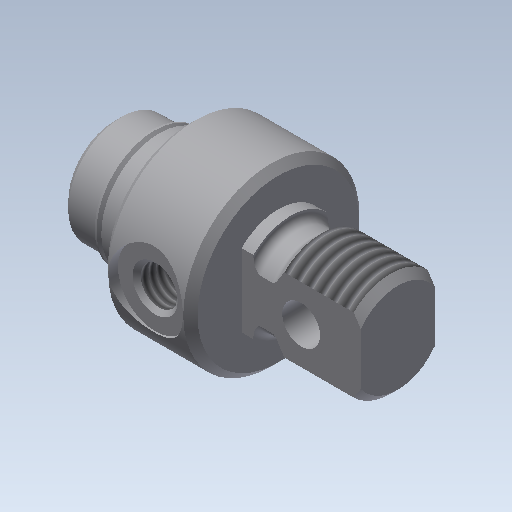
# Autodesk Inventor part: 01P0000_rear_head
Saved by Autodesk Inventor 2020 (Build 240168000, 168)
## iProperties
Created: 2020-01-07
Part Number: 01P0000_rear_head
Material: Generic
Catalog Web Link: www.cadenas.de
Description: Rear Head-Original Line - Standard Air Cylinders
Vendor: BIMBA
Document SubType Name: Modeling
Designer: psadmin
Manufacturer: BIMBA
Mass: 3.86005 g
Surface Area: 22.3376 cm^2
Volume: 3.86005 cm^3
Density: 1 g/cm^3
Appearance: PSOLRGB-211-211-211
Category: PARTsolutions
Company: BIMBA
PSOL_IDENT_0: {$CADENAS_DATA\23d-libs\bimba\bimba_brand\bimba_imperial\bimba_full_line\original_line_cylinders\sta
PSOL_IDENT_1: ndard_air_cylinders\rear_head.prj},239 {VTYP=3D},{NB=01P0000_rear_head},{LINA=01P0000_rear_head},{NN=
PSOL_IDENT_2: Rear Head},{DATE=23.12.2019 10:40:48},{GEOMDATE=15.10.2019 12:00:43},{VERSION=},{LINEID=20},{WBVAR=M
PSOL_IDENT_3: NT,ACTING,DER,Q,T1,T2,T3,T4,TRIM,Y,K,MB,CUSH,FBON},{WBNUMERIC=TRIM,MB,CUSH}  {NB=01P0000_rear_head},
PSOL_IDENT_4: {LINA=01P0000_rear_head},{KT=DUMMY},{PN=01P0000},{BORE=0.43750},{BOREPN=01},{MNT=P},{MNTALG='' , 'Fr
PSOL_IDENT_5: ont Nose' , 'P' , 'Rear Pivot' , 'DX' , 'Double End' , 'BR' , 'Rear Block' , 'BRT' , 'Rear Trunnion'
PSOL_IDENT_6: },{ACTING=},{ACTINGALG= '' , 'Single Acting' },{DER=},{DERALG= '' , 'Standard' },{Q=},{T1=},{T2=},{T
PSOL_IDENT_7: 3=},{T4=},{TRIM=0},{Y=},{K=},{KALG= '', 'without K', 'K', 'with K' },{MB=0},{A1=1.1880},{A1N=0.5000}
PSOL_IDENT_8: ,{A1P=1.1880},{A1B=0.8120},{A1S=0.0000},{A2=0.188},{A2N=0.1880},{A3=0.0200},{D1=0.7380},{D1N=0.4855}
PSOL_IDENT_9: ,{D1P=0.7380},{D1B=0.4855},{D2=0.4465},{C1=0.0300},{C2=0.0300},{NDM=0.1900},{TAB=UNF},{NDMDP=0.2000}
PSOL_IDENT_10: ,{D3=0.1600},{A4=0.1880},{A5=0.3700},{D4=0.0000},{A6=0.0000},{A7=0.5000},{A8=0.1250},{D5=0.4855},{D6=
PSOL_IDENT_11: 0.1875},{A9=0.6250},{NDM2=0.4375},{TAB2=UNF},{C11=0.0300},{C22=0.0000},{C33=0.0300},{C44=0.0300},{A1
PSOL_IDENT_12: 0=0.3095},{A11=0.0000},{NDM3=0.1900},{NDM3N=0.1900},{NDM3B=0.1900},{TAB3=UNF},{TAB3N=UNF},{TAB3B=UNF
PSOL_IDENT_13: },{A12=0.5},{A12N=0.5000},{A12B=0.4680},{A13=0.9380},{D7=0.1590},{D8=0.4350},{A14=0.0500},{A15=0.077
PSOL_IDENT_14: 5},{D9=0.3600},{R1=0.0315},{X1=0.0000},{X2=0.0000},{CX=0.0000},{CC=0.0000},{CON=1},{S1=0.7500},{DB=0
PSOL_IDENT_15: .1562},{X1B=0.2500},{X2B=0.0620},{A8B=0.1250},{A9B=0.5620},{MODEL=1},{NDM4=0.1640},{TAB4=UNC},{NDM4D
PSOL_IDENT_16: P=0.2500},{BC=0.7500},{B1=0.5620},{B2=0.2500},{B3=0.3740},{ON=0},{ON2=1},{G1=0.0000},{G2=0.0000},{G3=
PSOL_IDENT_17: 0.0000},{G4=0.0000},{GD=0.0000},{G5=0.0000},{G6=0.0000},{RON=0},{H1=0.0000},{H2=0.0000},{H3=0.0000},
PSOL_IDENT_18: {H4=0.0000},{H5=0.0000},{H6=0.0000},{F=0.0000},{PNUT=0.7380},{CUSH=0},{CC11=0.000},{CC111=0.0000},{C
PSOL_IDENT_19: C22=0.0000},{CC33=0.0000},{CC44=0.0000},{CC55=0.0000},{CD1=0.0000},{CD2=0.0000},{CD3=0.0000},{CNDM3=
PSOL_IDENT_20: 0.0000},{CTAB3=0.0000},{OLEN=0.9380},{OD=0.2185},{STDIS=0.0000},{STDIS1=0.0000},{BUSHCON=D-8597},{BU
PSOL_IDENT_21: SHL=0.3120},{FBON=0},{LCD=0.0000}
NN: Rear Head
NT: Original Line - Standard Air Cylinders
NB: 01P0000_rear_head
NBSYN: $PN._rear_head
LINA: 01P0000_rear_head
PN: 01P0000
BORE: 0.4375
BOREPN: 01
MNT: Rear Pivot
MNTALG: '' , 'Front Nose' , 'P' , 'Rear Pivot' , 'DX' , 'Double End' , 'BR' , 'Rear Block' , 'BRT' , 'Rear Trunnion'
ACTING: Single Acting
DER: Standard
Q: Without Side Ported Rear Head
T1: without T1
T2: without T2
T3: without T3
T4: without T4
TRIM: 0
Y: without Pivot Bushing
K: without K
MB: 0
A1N: 0.5
A1P: 1.188
A1B: 0.812
A1S: 0
A2N: 0.188
A3: 0.02
D1N: 0.4855
D1P: 0.738
D1B: 0.4855
D2: 0.4465
C1: 0.03
C2: 0.03
TAB: UNF
NDMDP: 0.2
D3: 0.16
A4: 0.188
A5: 0.37
D4: 0
A6: 0
A7: 0.5
A8: 0.125
D5: 0.4855
D6: 0.1875
A9: 0.625
NDM2: 0.4375
TAB2: UNF
C11: 0.03
C22: 0
C33: 0.03
C44: 0.03
A10: 0.3095
A11: 0
NDM3N: 0.19
NDM3B: 0.19
TAB3N: UNF
TAB3B: UNF
A12N: 0.5
A12B: 0.468
A13: 0.938
D7: 0.159
D8: 0.435
A14: 0.05
A15: 0.0775
D9: 0.36
R1: 0.0315
X1: 0
X2: 0
CX: 0
CC: 0
S1: 0.75
DB: 0.1562
X1B: 0.25
X2B: 0.062
A8B: 0.125
A9B: 0.562
NDM4: 0.164
TAB4: UNC
NDM4DP: 0.25
BC: 0.75
B1: 0.562
B2: 0.25
B3: 0.374
G1: 0
G2: 0
G3: 0
G4: 0
GD: 0
G5: 0
G6: 0
H2: 0
H3: 0
F: 0
CUSH: 0
CC111: 0
CC22: 0
CC33: 0
CC44: 0
CC55: 0
CD1: 0
CD2: 0
CD3: 0
CNDM3: 0
CTAB3: 0.0000
OD: 0.2185
STDIS1: 0
BUSHCON: D-8597
BUSHL: 0.312
FBON: 0
LCD: 0
SUPPLIER: BIMBA
ARTICLENO: 01P0000_rear_head
BOMINFO: 01P0000_rear_head
CREATOR: CADENAS GmbH
Title: 01P0000_rear_head
Author: Cadenas PARTsolutions
Comments: Original Line - Standard Air Cylinders
Autodesk Inventor part; units mm, degrees
ref_plane "YZ Plane" through (0, 0, 0) normal (1, 0, 0) x (0, 1, 0)
ref_plane "XZ Plane" through (0, 0, 0) normal (0, 1, 0) x (-1, 0, 0)
ref_plane "XY Plane" through (0, 0, 0) normal (0, 0, 1) x (1, 0, 0)
sketch "Sketch_8" plane through (0, 0, 0) normal (0, 0, 1) x (1, 0, 0)
  line L0 (17.4752, 0) -> (0, 0)
  line L1 (0, 0) -> (0, 4.9085)
  line L2 (0, 4.9085) -> (0.762, 5.6706)
  line L3 (0.762, 5.6706) -> (3.7592, 5.6706)
  line L4 (3.7592, 5.6706) -> (4.2672, 5.1626)
  line L5 (4.2672, 5.1626) -> (4.7752, 5.1626)
  line L6 (4.7752, 5.1626) -> (4.7752, 6.1659)
  line L7 (4.7752, 6.1659) -> (7.9502, 6.1659)
  line L8 (7.9502, 6.1659) -> (7.9502, 8.6106)
  line L9 (7.9502, 8.6106) -> (8.7122, 9.3726)
  line L10 (8.7122, 9.3726) -> (16.7132, 9.3726)
  line L11 (16.7132, 9.3726) -> (17.4752, 8.6106)
  line L12 (17.4752, 8.6106) -> (17.4752, 0)
  line L13 (17.4752, 0) -> (0, 0)
  constraints: 28 end point
revolve "Revolution1" add sketch "Sketch_8" angle 360 about axis through (17.4752, 0, 0) along (1, 0, 0)
sketch "Sketch_15" plane through (0, 0, 0) normal (0, 0, 1) x (1, 0, 0)
  line L0 (30.1752, 0) -> (17.4752, 0)
  line L1 (17.4752, 0) -> (17.4752, 5.5245)
  line L2 (17.4752, 5.5245) -> (18.7452, 5.5245)
  line L3 (18.7452, 5.5245) -> (18.7452, 5.3721)
  arc A0 (18.7452, 5.3721) -> (19.5453, 4.572) centre (19.5453, 5.3721) ccw
  line L4 (19.5453, 4.572) -> (20.7137, 4.572)
  arc A1 (20.7137, 4.572) -> (21.2166, 4.7498) centre (20.7137, 5.3721) ccw
  line L5 (21.2166, 4.7498) -> (21.2795, 4.8006)
  line L6 (21.2795, 4.8006) -> (22.0351, 5.5563)
  line L7 (22.0351, 5.5563) -> (29.4196, 5.5563)
  line L8 (29.4196, 5.5563) -> (30.1752, 4.8006)
  line L9 (30.1752, 4.8006) -> (30.1752, 0)
  line L10 (30.1752, 0) -> (17.4752, 0)
  constraints: 22 end point, 4 point on circle, 2 centre point
revolve "Revolution2" add sketch "Sketch_15" angle 360 about axis through (30.1752, 0, 0) along (1, 0, 0)
thread "Thread1" size "7/16-20 UNF" class "2A" standard "ANSI Unified Screw Threads" full length
sketch "Sketch_9" plane through (30.1752, 0, 0) normal (1, 0, 0) x (0, 0, -1)
  line L0 (-18.7452, -37.4904) -> (18.7452, -37.4904)
  line L1 (18.7452, -37.4904) -> (18.7452, 37.4904)
  line L2 (18.7452, 37.4904) -> (-18.7452, 37.4904)
  line L3 (-18.7452, 37.4904) -> (-18.7452, -37.4904)
  line L4 (-3.9306, -18.7452) -> (3.9306, -18.7452)
  line L5 (3.9306, -18.7452) -> (3.9306, 18.7452)
  line L6 (3.9306, 18.7452) -> (-3.9306, 18.7452)
  line L7 (-3.9306, 18.7452) -> (-3.9306, -18.7452)
  constraints: 16 end point
extrude "Extrusion1" cut sketch "Sketch_9" against normal blind 12.7
sketch "Sketch4" plane through (0, 0, 0) normal (-1, 0, 0) x (0, 0, 1)
  point P0 (0, 0)
hole "Hole1" at (0, 0, 0) direction (1, 0, 0) diameter 4.7625 depth 17.4625 tip angle 120
sketch "Sketch_16" plane through (0, 0, 0) normal (0, 1, 0) x (-1, 0, 0)
  line L0 (-12.7, 9.3726) -> (-12.7, 0)
  line L1 (-12.7, 0) -> (-14.6837, 0)
  line L2 (-14.6837, 0) -> (-14.6837, 7.9273)
  line L3 (-14.6837, 7.9273) -> (-15.113, 8.3566)
  line L4 (-15.113, 8.3566) -> (-16.6624, 8.3566)
  line L5 (-16.6624, 8.3566) -> (-16.6624, 9.3726)
  line L6 (-16.6624, 9.3726) -> (-12.7, 9.3726)
  line L7 (-12.7, 9.3726) -> (-12.7, 0)
  constraints: 16 end point
revolve "Revolution3" cut sketch "Sketch_16" angle 360 about axis through (12.7, 0, 9.3726) along (0, 0, 1)
thread "Thread2" size "10-32 UNF" class "2B" standard "ANSI Unified Screw Threads" length 5.5461
sketch "Sketch_24" plane through (0, 0, 0) normal (0, 0, 1) x (1, 0, 0)
  line L0 (4.7752, 0) -> (4.2672, 0)
  line L1 (4.0665, 6.1659) -> (4.0665, 6.0817)
  line L2 (4.0665, 6.0817) -> (4.6636, 5.4846)
  arc A0 (4.6636, 5.305) -> (4.6636, 5.4846) centre (4.5738, 5.3948) ccw
  line L3 (4.6636, 5.305) -> (4.5212, 5.1626)
  line L4 (4.5212, 5.1626) -> (4.2672, 5.1626)
  line L5 (4.2672, 5.1626) -> (4.2672, 4.9085)
  line L6 (4.2672, 4.9085) -> (4.7752, 4.9085)
  line L7 (4.7752, 4.9085) -> (4.7752, 5.6603)
  line L8 (4.7752, 5.6603) -> (4.2697, 6.1659)
  line L9 (4.2697, 6.1659) -> (4.0665, 6.1659)
  constraints: 20 end point, 2 point on circle, 1 centre point
revolve "Revolution4" add sketch "Sketch_24" angle 360 about axis through (4.7752, 0, 0) along (1, 0, 0)
sketch "Sketch_43" plane through (0, 0, 0) normal (0, 0, 1) x (1, 0, 0)
  circle A0 centre (23.8252, 0) radius 2.0193
  constraints: 1 centre point
extrude "Extrusion2" cut sketch "Sketch_43" along normal mid plane 11.7919
ref_plane "1_XY" through (18.7452, 0, 0) normal (1, 0, 0) x (0, 0, -1)
ref_plane "1_YZ" through (18.7452, 0, 0) normal (0, 0, -1) x (0, 1, 0)
ref_plane "1_ZX" through (18.7452, 0, 0) normal (0, 1, 0) x (1, 0, 0)
ref_plane "c1_XY" through (17.4752, 5.5245, 0) normal (0, 0, 1) x (1, 0, 0)
ref_plane "c1_YZ" through (17.4752, 5.5245, 0) normal (1, 0, 0) x (0, 1, 0)
ref_plane "c1_ZX" through (17.4752, 5.5245, 0) normal (0, 1, 0) x (0, 0, 1)
ref_plane "c2_XY" through (17.4752, -5.5245, 0) normal (0, 0, 1) x (1, 0, 0)
ref_plane "c2_YZ" through (17.4752, -5.5245, 0) normal (1, 0, 0) x (0, 1, 0)
ref_plane "c2_ZX" through (17.4752, -5.5245, 0) normal (0, 1, 0) x (0, 0, 1)
ref_plane "cc1_XY" through (17.4752, 0, 0) normal (0, 0, 1) x (1, 0, 0)
ref_plane "cc1_YZ" through (17.4752, 0, 0) normal (1, 0, 0) x (0, 1, 0)
ref_plane "cc1_ZX" through (17.4752, 0, 0) normal (0, 1, 0) x (0, 0, 1)
ref_plane "cc2_XY" through (18.7452, 0, 0) normal (0, 0, 1) x (1, 0, 0)
ref_plane "cc2_YZ" through (18.7452, 0, 0) normal (1, 0, 0) x (0, 1, 0)
ref_plane "cc2_ZX" through (18.7452, 0, 0) normal (0, 1, 0) x (0, 0, 1)
ref_plane "lovra1_XY" through (25.4, 0, 0) normal (1, 0, 0) x (0, 0, -1)
ref_plane "lovra1_YZ" through (25.4, 0, 0) normal (0, 0, -1) x (0, 1, 0)
ref_plane "lovra1_ZX" through (25.4, 0, 0) normal (0, 1, 0) x (1, 0, 0)
ref_plane "lovra2_XY" through (25.4, 4.699, 0) normal (1, 0, 0) x (0, 0, -1)
ref_plane "lovra2_YZ" through (25.4, 4.699, 0) normal (0, 0, -1) x (0, 1, 0)
ref_plane "lovra2_ZX" through (25.4, 4.699, 0) normal (0, 1, 0) x (1, 0, 0)
ref_plane "lovra21_XY" through (0, 0, 5.2705) normal (1, 0, 0) x (0, 0, -1)
ref_plane "lovra21_YZ" through (0, 0, 5.2705) normal (0, 0, -1) x (0, 1, 0)
ref_plane "lovra21_ZX" through (0, 0, 5.2705) normal (0, 1, 0) x (1, 0, 0)
ref_plane "lovra22_XY" through (0, 0, -5.2705) normal (1, 0, 0) x (0, 0, -1)
ref_plane "lovra22_YZ" through (0, 0, -5.2705) normal (0, 0, -1) x (0, 1, 0)
ref_plane "lovra22_ZX" through (0, 0, -5.2705) normal (0, 1, 0) x (1, 0, 0)
ref_plane "lovra3_XY" through (25.4, -4.699, 0) normal (1, 0, 0) x (0, 0, -1)
ref_plane "lovra3_YZ" through (25.4, -4.699, 0) normal (0, 0, -1) x (0, 1, 0)
ref_plane "lovra3_ZX" through (25.4, -4.699, 0) normal (0, 1, 0) x (1, 0, 0)
ref_plane "olen_XY" through (23.8252, 0, 0) normal (1, 0, 0) x (0, 0, -1)
ref_plane "olen_YZ" through (23.8252, 0, 0) normal (0, 0, -1) x (0, 1, 0)
ref_plane "olen_ZX" through (23.8252, 0, 0) normal (0, 1, 0) x (1, 0, 0)
ref_plane "p1_XY" through (30.1752, 0, 3.9306) normal (1, 0, 0) x (0, 0, -1)
ref_plane "p1_YZ" through (30.1752, 0, 3.9306) normal (0, 0, -1) x (0, 1, 0)
ref_plane "p1_ZX" through (30.1752, 0, 3.9306) normal (0, 1, 0) x (1, 0, 0)
ref_plane "p2_XY" through (30.1752, 0, -3.9306) normal (1, 0, 0) x (0, 0, -1)
ref_plane "p2_YZ" through (30.1752, 0, -3.9306) normal (0, 0, -1) x (0, 1, 0)
ref_plane "p2_ZX" through (30.1752, 0, -3.9306) normal (0, 1, 0) x (1, 0, 0)
ref_plane "port_XY" through (12.7, 0, 0) normal (0, 0, 1) x (1, 0, 0)
ref_plane "port_YZ" through (12.7, 0, 0) normal (1, 0, 0) x (0, 1, 0)
ref_plane "port_ZX" through (12.7, 0, 0) normal (0, 1, 0) x (0, 0, 1)
ref_plane "port2_XY" through (30.1752, 0, 0) normal (1, 0, 0) x (0, 0, -1)
ref_plane "port2_YZ" through (30.1752, 0, 0) normal (0, 0, -1) x (0, 1, 0)
ref_plane "port2_ZX" through (30.1752, 0, 0) normal (0, 1, 0) x (1, 0, 0)
ref_plane "thd1_XY" through (30.1752, 0, 5.5563) normal (1, 0, 0) x (0, 0, -1)
ref_plane "thd1_YZ" through (30.1752, 0, 5.5563) normal (0, 0, -1) x (0, 1, 0)
ref_plane "thd1_ZX" through (30.1752, 0, 5.5563) normal (0, 1, 0) x (1, 0, 0)
ref_plane "thd2_XY" through (30.1752, 0, -5.5563) normal (1, 0, 0) x (0, 0, -1)
ref_plane "thd2_YZ" through (30.1752, 0, -5.5563) normal (0, 0, -1) x (0, 1, 0)
ref_plane "thd2_ZX" through (30.1752, 0, -5.5563) normal (0, 1, 0) x (1, 0, 0)
ref_plane "to_mounting_bracket_XY" through (17.4752, 0, 0) normal (1, 0, 0) x (0, 0, -1)
ref_plane "to_mounting_bracket_YZ" through (17.4752, 0, 0) normal (0, 0, -1) x (0, 1, 0)
ref_plane "to_mounting_bracket_ZX" through (17.4752, 0, 0) normal (0, 1, 0) x (1, 0, 0)
ref_plane "to_nut_XY" through (18.7452, 0, 0) normal (1, 0, 0) x (0, 0, -1)
ref_plane "to_nut_YZ" through (18.7452, 0, 0) normal (0, 0, -1) x (0, 1, 0)
ref_plane "to_nut_ZX" through (18.7452, 0, 0) normal (0, 1, 0) x (1, 0, 0)
ref_plane "to_pin_XY" through (23.8252, 0, 0) normal (0, 0, 1) x (1, 0, 0)
ref_plane "to_pin_YZ" through (23.8252, 0, 0) normal (1, 0, 0) x (0, 1, 0)
ref_plane "to_pin_ZX" through (23.8252, 0, 0) normal (0, 1, 0) x (0, 0, 1)
ref_plane "to_screw_XY" through (12.7, 0, 0) normal (0, 1, 0) x (1, 0, 0)
ref_plane "to_screw_YZ" through (12.7, 0, 0) normal (1, 0, 0) x (0, 0, -1)
ref_plane "to_screw_ZX" through (12.7, 0, 0) normal (0, 0, -1) x (0, 1, 0)
ref_plane "to_tube_XY" through (4.2672, 0, 0) normal (1, 0, 0) x (0, 0, -1)
ref_plane "to_tube_YZ" through (4.2672, 0, 0) normal (0, 0, -1) x (0, 1, 0)
ref_plane "to_tube_ZX" through (4.2672, 0, 0) normal (0, 1, 0) x (1, 0, 0)
body "Solid1"
